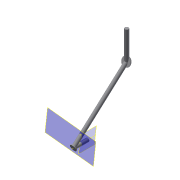
# Autodesk Inventor part: cellSTORM_lightpath
Saved by Autodesk Inventor 2019.4 (Build 234330000, 330)
## iProperties
Created: 2020-04-25
Part Number: cellSTORM_lightpath
Material: Generic
Document SubType Name: Modeling
Designer: diederichbenedict
Density: 1 g/cm^3
Appearance: Default
Mass: 3.01644 g
Surface Area: 25.0036 cm^2
Volume: 3.01644 cm^3
Author: diederichbenedict
Autodesk Inventor part; units mm, degrees
ref_plane "YZ Plane" through (0, 0, 0) normal (1, 0, 0) x (0, 1, 0)
ref_plane "XZ Plane" through (0, 0, 0) normal (0, 1, 0) x (-1, 0, 0)
ref_plane "XY Plane" through (0, 0, 0) normal (0, 0, 1) x (1, 0, 0)
ref_plane "Work Plane1" through (-18.0552, 1.9841, 10) normal (0, 0, -1) x (-0.9940164, 0.109231, 0)
ref_plane "Work Plane4" through (0, 0, 10) normal (-0.9940164, 0.109231, 0) x (-0.109231, -0.9940164, 0)
ref_plane "Work Plane3" through (-40.2485, 19.0101, 10) normal (-0.9940164, 0.109231, 0) x (-0.109231, -0.9940164, 0)
sketch "Sketch1" plane through (0, 0, 10) normal (-1, 0, 0) x (0, -1, 0)
  line L0 (0, -10) -> (0, 0)
  line L1 (0, 0) -> (-56.5685, -56.5685)
  line L2 (-7.1094, 2.5876) -> (7.1094, -2.5876)
  line L3 (-56.5685, -56.5685) -> (-86.5685, -56.5685)
  dimension "d0" = 10
  dimension "d1" = 80
  dimension "d2" = 45
  dimension "d6" = 70
  dimension "d23" = 30
  constraints: 8 end point, 1 horizontal, 1 midpoint, 1 vertical
  measures "d0" distance of L0.end L0.start
  measures "d1" distance of L0.end L1.end
  measures "d2" angle of L1 L0
  measures "d6" angle of L2 L0
  measures "d23" distance of L1.end L3.end
ref_plane "Work Plane7" through (-18.0552, 1.9841, 10) normal (0, 0, -1) x (-0.9940164, 0.109231, 0)
sketch "Sketch3" plane through (-18.0552, 1.9841, 10) normal (0, 0, -1) x (-0.9940164, 0.109231, 0)
  circle A0 centre (-18.1638, 0) radius 11.5 projected
  circle A1 centre (-18.1638, 0) radius 2.5
  point P0 (-18.1638, 0)
  dimension "d7" = 5
  constraints: 1 centre point, 1 coincident
  measures "d7" diameter of A1
sweep "Sweep1" add profiles "Sketch3" path "Sketch1" path curves L0 L1 L3 contours A1
sketch "Sketch7" plane through (0, 0, 10) normal (-1, 0, 0) x (0, -1, 0)
  line L0 (0, 0) -> (0, 0) projected
  line L1 (0, 0) -> (0, 0) projected
  line L2 (2.5, -10) -> (-2.5, -10) projected
  line L3 (0, 0) -> (0, 0) projected
  line L4 (0, 0) -> (0, 0) projected
  line L5 (2.5, -10) -> (2.5, 6.0355) projected
  line L6 (-2.5, -10) -> (-2.5, -6.0355) projected
  line L7 (-2.5, -6.0355) -> (0, 0) projected
  line L8 (0, -10) -> (0, 10)
  line L9 (4.554, -1.8863) -> (-22.0344, 9.1269)
  line L10 (-22.0344, 9.1269) -> (3.9261, 19.2345)
  line L11 (3.9261, 19.2345) -> (13.0438, 2.8333)
  line L12 (13.0438, 2.8333) -> (4.554, -1.8863)
  line L13 (-48.3403, -54.2978) -> (-48.6823, -53.3019)
  line L14 (-73.7647, -67.98) -> (-66.6763, -71.8283)
  line L15 (-66.6763, -71.8283) -> (-47.7403, -64.4229)
  line L16 (-47.7403, -64.4229) -> (-48.3403, -54.2978)
  line L17 (-55.533, -59.0685) -> (-56.5685, -56.5685) projected
  line L18 (-48.6823, -53.3019) -> (-76.2479, -64.72)
  line L19 (-76.2479, -64.72) -> (-73.7647, -67.98)
  point P0 (-65.0552, -65.9873)
  constraints: 22 end point, 2 perpendicular, 2 point on line, 1 vertical, 2 other
extrude "Extrusion4" cut sketch "Sketch7" along normal mid plane 10 contours L9 L10 L11 L12 | L16 L15 L14 L19 L18 L13
sketch "Sketch8" plane through (0, 0, 10) normal (0, -0.3826834, 0.9238795) x (1, 0, 0)
  ellipse E0 centre (0, 0) end of major axis (0, 2.706) minor radius 2.5 (2.5, 0) -> (-2.5, 0) ccw projected
  ellipse E1 centre (0, 0) end of major axis (0, -2.706) minor radius 2.5 (-2.5, 0) -> (2.5, 0) ccw projected
  circle A0 centre (0, 0) radius 4.3056
  point P0 (0, -3.8268)
  constraints: 1 centre point, 1 coincident, 2 other
extrude "Extrusion5" add sketch "Sketch8" against normal blind 1 contours E1 E0 | A0
sketch "Sketch9" plane through (0.4945, 62.5722, -49.0554) normal (0, -0.3826834, -0.9238795) x (-1, 0, 0)
  ellipse E0 centre (0.4945, -6.4984) end of major axis (0.4945, -13.0312) minor radius 2.5 (2.9945, -6.4984) -> (-2.0055, -6.4984) ccw projected
  ellipse E1 centre (0.4945, -6.4984) end of major axis (0.4945, 0.0345) minor radius 2.5 (-2.0055, -6.4984) -> (2.9945, -6.4984) ccw projected
  circle A0 centre (0.4945, -6.4984) radius 10.9648
  point P0 (0.4945, -76.5819)
  constraints: 1 centre point, 1 coincident, 2 other
extrude "Extrusion6" add sketch "Sketch9" against normal blind 1 contours E1 E0 | A0
ref_plane "Work Plane2" through (-1.6385, -14.9102, 10) normal (0, 0, 1) x (0.9940164, -0.109231, 0)
body "Solid1"
